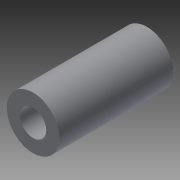
# Autodesk Inventor part: Separador SAV (V2)
Saved by Autodesk Inventor 2014 (Build 180170000, 170)
## iProperties
Created: 2014-12-03
Part Number: Separador SAV (V2)
Material: Generic
Document SubType Name: Modeling
Designer: Rubén
Density: 1 g/cm^3
Appearance: Default
Author: Rubén
Autodesk Inventor part; units mm, degrees
ref_plane "YZ Plane" through (0, 0, 0) normal (1, 0, 0) x (0, 1, 0)
ref_plane "XZ Plane" through (0, 0, 0) normal (0, 1, 0) x (-1, 0, 0)
ref_plane "XY Plane" through (0, 0, 0) normal (0, 0, 1) x (1, 0, 0)
sketch "Sketch1" plane through (0, 0, 0) normal (0, 0, 1) x (1, 0, 0)
  circle A0 centre (0, 0) radius 3
  circle A1 centre (0, 0) radius 1.5
  dimension "d0" = 6
  dimension "d1" = 3
  constraints: 2 centre point, 2 coincident
  measures "d0" diameter of A0
  measures "d1" diameter of A1
extrude "Extrusion1" add sketch "Sketch1" along normal blind 13
body "Solid1"
